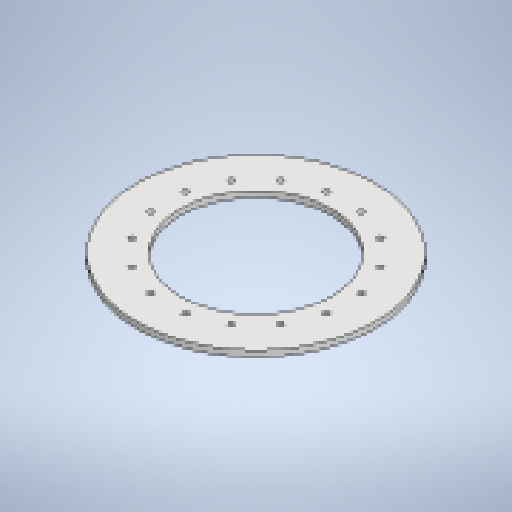
# Autodesk Inventor part: ДМФ 025 кольцо прижимное корма наружное v2.0
Saved by Autodesk Inventor 2025 (Build 290162010, 162A)
## iProperties
Created: 2024-04-23
Part Number: ДМФ 025 кольцо прижимное корма наружное v2.0
Material: Generic
Document SubType Name: Sheet Metal
Designer: admin
Stock Number: ДМФ 025 кольцо прижимное корма наружное
Density: 1 g/cm^3
Flat Pattern Width: 60 cm
Flat Pattern Length: 60 cm
Flat Pattern Area: 3600 cm^2
Sheet Metal Rule: Default
Sheet Metal Width: 600,000 mm
Sheet Metal Length: 600,000 mm
Sheet Metal Area: 360000,000 mm^2
Appearance: Default
Author: admin
Autodesk Inventor part; units mm, degrees
ref_plane "YZ Plane" through (0, 0, 0) normal (1, 0, 0) x (0, 1, 0)
ref_plane "XZ Plane" through (0, 0, 0) normal (0, 1, 0) x (-1, 0, 0)
ref_plane "XY Plane" through (0, 0, 0) normal (0, 0, 1) x (1, 0, 0)
sketch "Sketch1" plane through (0, 0, 0) normal (0, 0, 1) x (1, 0, 0)
  circle A0 centre (0, 0) radius 190
  circle A1 centre (0, 0) radius 300
  point P0 (0, 225)
  dimension "d41" = 600
  dimension "d42" = 380
  constraints: 2 centre point, 2 coincident, 1 vertical alignment
  measures "d41" diameter of A1
  measures "d42" diameter of A0
extrude "Extrusion1" add sketch "Sketch1" along normal blind 15
sketch "Sketch3" plane through (0, 0, 0) normal (0, 0, 1) x (1, 0, 0)
  circle A0 centre (0, 0) radius 190 construction
  circle A1 centre (0, 0) radius 300 construction
  circle A2 centre (0, 0) radius 300 construction
  line L0 (0, 0) -> (0, -300) construction
  line L1 (0, 0) -> (58.5271, -294.2356) construction
  line L2 (47.602, -239.3116) -> (40.1886, -202.0418) construction
  circle A3 centre (43.8953, -220.6767) radius 7
  circle A4 centre (0, 0) radius 225 construction
  dimension "d43" = 450
  dimension "d20" = 11.25
  dimension "d21" = 14
  constraints: 6 end point, 2 point on circle, 2 point on line, 1 centre point, 1 coincident, 1 midpoint, 1 vertical, 3 other
  measures "d20" angle of L1 L0
  measures "d21" diameter of A3
extrude "Extrusion3" cut sketch "Sketch3" along normal through all
pattern_circular "Circular Pattern2" count 16 over 360 about axis through (0, 0, 0) along (0, 0, -1) of "Extrusion3"
equation "\"BendRadius\" = Thickness"
equation "\"BendReliefWidth\" = Thickness"
equation "\"BendReliefDepth\" = 0.5 * Thickness"
equation "\"CornerReliefSize\" = 4 * Thickness"
equation "\"MinimumRemnant\" = 2 * Thickness"
equation "\"TransitionRadius\" = BendRadius"
equation "\"JacobiRadiusSize\" = BendRadius"
equation "\"GapSize\" = Thickness"
equation "\"Thickness\" = 3"
body "Solid1"
